square (Autodesk Fusion 360 design; units mm, degrees)
Autodesk Fusion 360 part; units mm, degrees
sketch "Sketch1" plane through (0, 0, 0) normal (0, 0, 1) x (1, 0, 0)
  line L0 (-5.85, 5.85) -> (5.85, 5.85)
  line L1 (5.85, 5.85) -> (5.85, -5.85)
  line L2 (5.85, -5.85) -> (-5.85, -5.85)
  line L3 (-5.85, -5.85) -> (-5.85, 5.85)
  line L4 (-5.85, 5.85) -> (5.85, -5.85) construction
  line L5 (5.85, 5.85) -> (-5.85, -5.85) construction
  line L6 (11.0385, 11.0385) -> (-11.0385, 11.0385)
  line L7 (-11.0385, 11.0385) -> (-11.0385, -11.0385)
  line L8 (-11.0385, -11.0385) -> (11.0385, -11.0385)
  line L9 (11.0385, -11.0385) -> (11.0385, 11.0385)
  line L10 (11.0385, 11.0385) -> (-11.0385, -11.0385) construction
  line L11 (-11.0385, 11.0385) -> (11.0385, -11.0385) construction
  dimension "d1" = 11.7
  constraint horizontal L0
  constraint perpendicular L0 L1
  constraint parallel L0 L2
  constraint parallel L1 L3
  constraint coincident L4 origin
  constraint coincident L5 origin
  constraint equal L0 L1
  constraint horizontal L6
  constraint perpendicular L6 L7
  constraint parallel L6 L8
  constraint parallel L7 L9
  constraint coincident L10 origin
  constraint coincident L11 origin
  measures "d1" distance of L0 L2
extrude "Extrude1" add sketch "Sketch1" against normal blind 10 makes body 1
extrude "Extrude2" add sketch "Sketch1" along normal blind 5 contours L0 L1 L2 L3 | L6 L7 L8 L9 bodies 1
extrude "Extrude3" add sketch "Sketch1" along normal blind 11 from surface at 5 contours L0 L1 L2 L3 bodies 1
chamfer "Chamfer1" distance 1 angle 45 1 faces at (1.95, -9.309, 5) on bodies 1
chamfer "Chamfer2" distance 1 angle 45 1 faces at (-1.95, 1.95, 0) on bodies 1
extrude "Extrude4" add sketch "Sketch1" along normal blind 22 separate body contours L0 L1 L2 L3 makes body 2
move_face "OffsetFaces1" offset 3.737 1 faces at (-1.95, 1.95, 22) on bodies 2
hidden bodies 1
